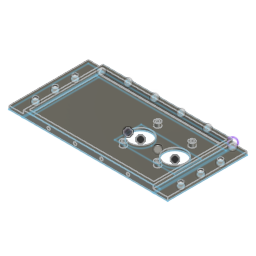
Side-Panel-120x60mmtemp (Autodesk Fusion 360 design; units mm, degrees)
part number: 2026-04-12-13-41-56-896
Autodesk Fusion 360 part; units mm, degrees
sketch "Sketch1" plane through (0, 0, 0) normal (0, 0, 1) x (1, 0, 0)
  line L0 (60, 30) -> (-60, 30)
  line L1 (-60, 30) -> (-60, -30)
  line L2 (-60, -30) -> (60, -30)
  line L3 (60, -30) -> (60, 30)
  line L4 (-50, 30) -> (-50, -30)
  line L5 (50, 30) -> (50, -30)
  circle A0 centre (-55, 15) radius 1.75
  circle A1 centre (-55, 0) radius 1.75
  circle A2 centre (-55, -15) radius 1.75
  circle A3 centre (55, 15) radius 1.75
  circle A4 centre (55, 0) radius 1.75
  circle A5 centre (55, -15) radius 1.75
  line L6 (-49, 25) -> (49, 25)
  line L7 (-49, -25) -> (49, -25)
  line L8 (-49, 30) -> (-49, 25)
  line L9 (-49, -25) -> (-49, -30)
  line L10 (49, 30) -> (49, 25)
  line L11 (49, -25) -> (49, -30)
  line L12 (-49, -25) -> (-49, 25)
  line L13 (-47, -25) -> (-47, 25)
  line L14 (49, -25) -> (49, 25)
  line L15 (47, -25) -> (47, 25)
  line L16 (45, 10) -> (0, 10)
  line L17 (0, 10) -> (0, -10)
  line L18 (0, -10) -> (45, -10)
  line L19 (45, -10) -> (45, 10)
  circle A6 centre (9.5, 0) radius 8.25
  circle A7 centre (35.5, 0) radius 8.25
  point P0 (22.5, 0)
  point P1 (9.5, 0)
  point P2 (35.5, 0)
  dimension "d25" = 16.5
  dimension "d26" = 16.5
  constraint horizontal L0
  constraint perpendicular L0 L1
  constraint parallel L0 L2
  constraint parallel L1 L3
  constraint coincident L2 L4.end
  constraint perpendicular L2 L4
  constraint coincident L0 L5.start
  constraint coincident L2 L5.end
  constraint perpendicular L2 L5
  constraint coincident L0 L8.start
  constraint coincident L2 L9.end
  constraint perpendicular L2 L9
  constraint coincident L2 L11.end
  constraint perpendicular L2 L11
  constraint perpendicular L6 L10
  constraint perpendicular L7 L11
  constraint collinear L8 L9
  constraint collinear L10 L11
  constraint coincident L7 L13.start
  constraint coincident L6 L13.end
  constraint perpendicular L6 L13
  constraint coincident L7 L15.start
  constraint coincident L6 L15.end
  constraint perpendicular L6 L15
  constraint horizontal L16
  constraint perpendicular L16 L17
  constraint parallel L16 L18
  constraint parallel L17 L19
  constraint coincident P1 A6.centre
  constraint coincident P2 A7.centre
  measures "d25" diameter of A6
  measures "d26" diameter of A7
extrude "Extrude1" add sketch "Sketch1" along normal blind 2.5 contours L0 L2 L3 L5 | L0 L2 L5 L10 L11 L14 | L0 L2 L4 L8 L9 L12 | L6 L7 L14 L15 | L0 L1 L2 L4 | L6 L7 L12 L13 makes body 1 at (54.7103, -23.915, 0) makes body 2 at (-54.7103, -23.915, 0)
sketch "Sketch2" plane through (0, 0, 2.5) normal (0, 0, 1) x (-1, 0, 0)
  circle A0 centre (-55, 0) radius 1.75
  circle A1 centre (55, -15) radius 1.75
  circle A2 centre (55, 15) radius 1.75
  circle A3 centre (55, 0) radius 1.75
  circle A4 centre (-55, 15) radius 1.75
  circle A5 centre (-55, -15) radius 1.75
  line L0 (-60, 30) -> (-60, -30)
  line L1 (-60, -30) -> (-49, -30)
  line L2 (60, -30) -> (60, 30)
  line L3 (-49, 30) -> (-60, 30)
  line L4 (-47, 25) -> (-49, 25)
  line L5 (-49, 25) -> (-49, 30)
  line L6 (-49, -30) -> (-49, -25)
  line L7 (-49, -25) -> (-47, -25)
  line L8 (49, -25) -> (49, -30)
  line L9 (49, -30) -> (60, -30)
  line L10 (60, 30) -> (49, 30)
  line L11 (49, 30) -> (49, 25)
  circle A6 centre (-9.5, -13) radius 1.2
  circle A7 centre (-35.5, -13) radius 1.2
  circle A8 centre (-35.5, 13) radius 1.2
  circle A9 centre (-9.5, 13) radius 1.2
  circle A10 centre (-9.5, 13) radius 2.25
  circle A11 centre (-35.5, 13) radius 2.25
  circle A12 centre (-9.5, -13) radius 2.25
  circle A13 centre (-35.5, -13) radius 2.25
  line L12 (-47, -25) -> (-47, 25)
  line L13 (49, 25) -> (47, 25)
  line L14 (47, 25) -> (47, -25)
  line L15 (47, -25) -> (49, -25)
  dimension "d28" = 2.4
  constraint concentric A9 A10
  measures "d28" diameter of A6
extrude "Extrude2" add sketch "Sketch1" along normal blind 5 separate body contours L0 L6 L8 L10 | L6 L7 L14 L15 | L2 L7 L9 L11 | L6 L7 L12 L13 makes body 3
sketch "Sketch3" plane through (0, -30, 0) normal (0, -1, 0) x (1, 0, 0)
  line L0 (-49, 0) -> (49, 0)
  line L1 (49, 0) -> (49, 5)
  line L2 (49, 5) -> (-49, 5)
  line L3 (-49, 5) -> (-49, 0)
  circle A0 centre (30, 2.5) radius 1.2
  circle A1 centre (10, 2.5) radius 1.2
  circle A2 centre (-10, 2.5) radius 1.2
  circle A3 centre (-30, 2.5) radius 1.2
extrude "Extrude3" cut sketch "Sketch3" against normal blind 3 contours A0 | A1 | A2 | A3 bodies 3
sketch "Sketch4" plane through (0, 30, 0) normal (0, 1, 0) x (-1, 0, 0)
  line L0 (-49, 0) -> (49, 0)
  line L1 (49, 0) -> (49, 5)
  line L2 (49, 5) -> (-49, 5)
  line L3 (-49, 5) -> (-49, 0)
  circle A0 centre (-30, 2.5) radius 1.2
  circle A1 centre (-10, 2.5) radius 1.2
  circle A2 centre (30, 2.5) radius 1.2
  circle A3 centre (10, 2.5) radius 1.2
  point P0 (-49, 2.5)
extrude "Extrude5" add sketch "Sketch2" along normal blind 3 separate body contours A10 | A11 | A12 | A13 makes body 4 at (7.2528, 13.1122, 4.5) makes body 5 at (7.2528, -12.8878, 4.5) makes body 6 at (33.2528, 13.1122, 4.5) makes body 7 at (33.2528, -12.8878, 4.5)
extrude "Extrude4" cut sketch "Sketch4" against normal blind 3 contours A0 | A1 | A2 | A3 bodies 3
chamfer "Chamfer1" distance 2.5 angle 45 2 edges at (0, 25, 5) (0, -25, 5) on bodies 3
extrude "Extrude6" add sketch "Sketch1" along normal blind 2 contours L6 L7 L13 L15 | L16 L17 L18 L19 bodies 1 2 3
